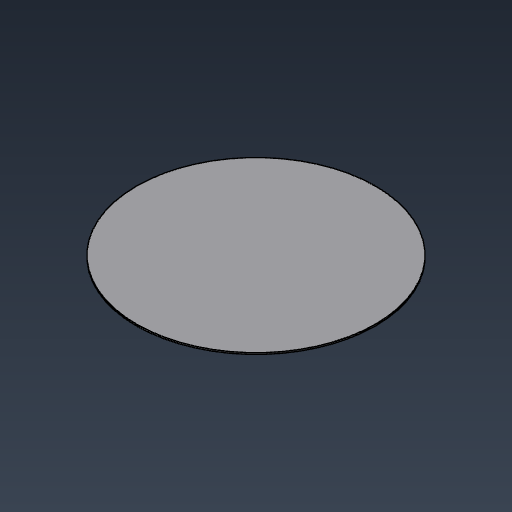
# Autodesk Inventor part: Papier 40mm
Saved by Autodesk Inventor 2023.1 (Build 271208000, 208)
## iProperties
Created: 2015-09-03
Part Number: Papier 40mm
Material: Allgemein
Document SubType Name: Modeling
Designer: ryll
Density: 1 g/cm^3
Appearance: Vorgabe
Mass: 0.314159 g
Surface Area: 25.4469 cm^2
Volume: 0.314159 cm^3
Author: ryll
Autodesk Inventor part; units mm, degrees
ref_plane "YZ Plane" through (0, 0, 0) normal (1, 0, 0) x (0, 1, 0)
ref_plane "XZ Plane" through (0, 0, 0) normal (0, 1, 0) x (-1, 0, 0)
ref_plane "XY Plane" through (0, 0, 0) normal (0, 0, 1) x (1, 0, 0)
sketch "Skizze1" plane through (0, 0, 0) normal (0, 0, 1) x (1, 0, 0)
  line L0 (-28, 0) -> (28, 0) projected
  line L1 (0, 28) -> (0, -28) projected
  circle A0 centre (0, 0) radius 20
  dimension "d6" = 40
  constraints: 2 midpoint, 1 centre point
  measures "d6" diameter of A0
extrude "Extrusion1" add sketch "Skizze1" along normal blind 0.25
